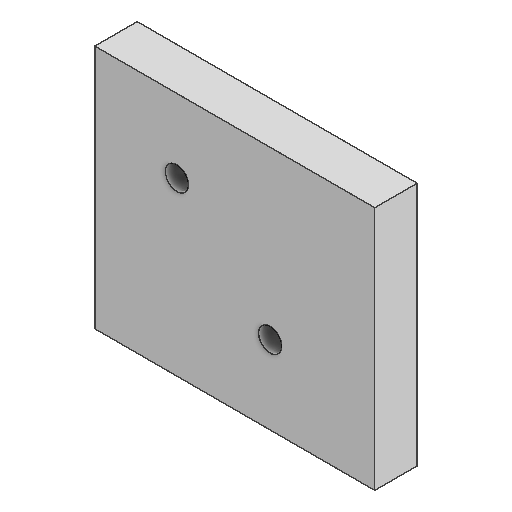
# Autodesk Inventor part: rearSwingarmBaseV1
Saved by Autodesk Inventor 2025 (Build 290162000, 162)
## iProperties
Created: 2025-01-09
Part Number: rearSwingarmBaseV1
Material: Generic
Document SubType Name: Modeling
Designer: derm
Density: 1 g/cm^3
Appearance: Default
Author: derm
Autodesk Inventor part; units mm, degrees
ref_plane "YZ Plane" through (0, 0, 0) normal (1, 0, 0) x (0, 1, 0)
ref_plane "XZ Plane" through (0, 0, 0) normal (0, 1, 0) x (-1, 0, 0)
ref_plane "XY Plane" through (0, 0, 0) normal (0, 0, 1) x (1, 0, 0)
sketch "Sketch1" plane through (0, 0, 0) normal (0, 0, 1) x (1, 0, 0)
  circle A0 centre (0, 0) radius 2.75
  circle A1 centre (-22, 22) radius 2.75
  circle A2 centre (0, 0) radius 11 construction
  circle A3 centre (-22, 22) radius 11 construction
  line L0 (-41.3602, 39.2963) -> (24.6813, 39.2963)
  line L1 (24.6813, 39.2963) -> (24.6813, -18.4462)
  line L2 (24.6813, -18.4462) -> (-41.3602, -18.4462)
  line L3 (-41.3602, -18.4462) -> (-41.3602, 39.2963)
  dimension "d0" = 5.5
  dimension "d1" = 5.5
  dimension "d2" = 22
  dimension "d3" = 22
  dimension "d4" = 22
  constraints: 8 end point, 4 centre point, 3 coincident, 2 parallel, 1 equal radius, 1 horizontal, 1 perpendicular
  measures "d0" diameter of A0
  measures "d1" diameter of A1
  measures "d2" horizontal distance of point (0, 0) A1.centre
  measures "d3" horizontal distance of point (0, 0) A1.centre
  measures "d4" diameter of A3
extrude "Extrusion1" add sketch "Sketch1" against normal blind 10
body "Solid1"
